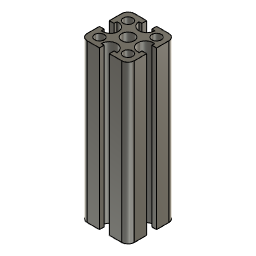
프로파일 2 v1 (Autodesk Fusion 360 design; units mm, degrees)
Autodesk Fusion 360 part; units mm, degrees
sketch "스케치1" plane through (0, 0, 0) normal (0, 0, 1) x (1, 0, 0)
  line L0 (-15, -11) -> (-15, -3.15)
  line L1 (-15, 3.15) -> (-15, 11)
  line L2 (15, 11) -> (15, 3.15)
  line L3 (15, -3.15) -> (15, -11)
  line L4 (-11, 15) -> (-3.15, 15)
  line L5 (3.15, 15) -> (11, 15)
  line L6 (11, -15) -> (3.15, -15)
  line L7 (-3.15, -15) -> (-11, -15)
  circle A0 centre (-9.075, 9.075) radius 3
  line L8 (-15.033, 3.15) -> (-12, 3.15)
  line L9 (-12, 9.075) -> (-12.075, 9.075)
  line L10 (-12, 4.9272) -> (-12, 3.15)
  circle A1 centre (0, 0) radius 4
  arc A2 (-15, 3.1902) -> (-15.033, 3.15) centre (-11.15, 0) ccw
  line L11 (-15.033, -3.15) -> (-12, -3.15)
  arc A3 (-15.033, -3.15) -> (-15, -3.1902) centre (-11.15, 0) ccw
  arc A4 (-12, -4.9272) -> (-12, 4.9272) centre (-11.15, 0) ccw
  line L12 (-5, 12) -> (-3.15, 12)
  arc A5 (-5, 12) -> (5, 12) centre (0, 12) ccw
  line L13 (-3.15, 15) -> (-3.15, 12)
  line L14 (3.15, 15) -> (3.15, 12)
  line L15 (3.15, 15) -> (3.15, 12)
  line L16 (12, 4.9272) -> (12, 3.15)
  arc A6 (12, 4.9272) -> (12, -4.9272) centre (11.15, 0) ccw
  line L17 (5, 12) -> (3.15, 12)
  line L18 (15, -11) -> (15, -3.15)
  arc A7 (15, -3.1902) -> (15.033, -3.15) centre (11.15, 0) ccw
  circle A8 centre (9.075, 9.075) radius 3
  line L19 (3.15, -15) -> (11, -15)
  arc A9 (15.033, 3.15) -> (15, 3.1902) centre (11.15, 0) ccw
  line L20 (15, 3.15) -> (15, 11)
  line L21 (-12, -3.15) -> (-12, -4.9272)
  line L22 (12, 3.15) -> (15, 3.15)
  line L23 (12, -3.15) -> (15, -3.15)
  line L24 (0, 0) -> (-20, 0)
  circle A10 centre (-9.075, -9.075) radius 3
  circle A11 centre (9.075, -9.075) radius 3
  line L25 (3.15, -15) -> (11, -15)
  line L26 (15, -11) -> (15, -3.15)
  line L27 (-15, -3.15) -> (-15, -11)
  line L28 (-15.033, -3.15) -> (-12, -3.15)
  arc A12 (5, -12) -> (-5, -12) centre (0, -12) ccw
  line L29 (15, -3.15) -> (15, -11)
  arc A13 (15, -3.1902) -> (15.033, -3.15) centre (11.15, 0) ccw
  arc A14 (-15.033, -3.15) -> (-15, -3.1902) centre (-11.15, 0) ccw
  line L30 (12, -4.9272) -> (12, -3.15)
  line L31 (12, -3.15) -> (15, -3.15)
  line L32 (-12, -4.9272) -> (-12, -3.15)
  line L33 (3.15, -15) -> (3.15, -12)
  line L34 (3.15, -15) -> (3.15, -12)
  line L35 (-5, -12) -> (-3.15, -12)
  line L36 (5, -12) -> (3.15, -12)
  line L37 (-3.15, -15) -> (-3.15, -12)
  line L38 (3.15, 12) -> (5, 12)
  line L39 (12, 4.9272) -> (12, 3.15)
  arc A15 (9.7416, 12) -> (12, 9.7416) centre (9.075, 9.075) ccw
  line L40 (-3.15, -12) -> (-3.15, -15)
  line L41 (3.15, -12) -> (3.15, -15)
  line L42 (3.15, -12) -> (3.15, -15)
  line L43 (3.15, -12) -> (5, -12)
  line L44 (3.15, -12) -> (5, -12)
  line L45 (12, -3.15) -> (12, -4.9272)
  line L46 (12, -4.9272) -> (12, -3.15)
  line L47 (12, -3.15) -> (12, -4.9272)
  arc A16 (6.075, -9.075) -> (8.4084, -6.15) centre (9.075, -9.075) ccw
  arc A17 (6.075, -9.075) -> (8.4084, -6.15) centre (9.075, -9.075) ccw
  arc A18 (6.075, -9.075) -> (8.4084, -6.15) centre (9.075, -9.075) ccw
  line L48 (-5, -12) -> (-3.15, -12)
  arc A19 (-8.4084, -6.15) -> (-12.075, -9.075) centre (-9.075, -9.075) ccw
  arc A20 (-11, 15) -> (-15, 11) centre (-11, 11) ccw
  arc A21 (15, 11) -> (11, 15) centre (11, 11) ccw
  arc A22 (11, -15) -> (15, -11) centre (11, -11) ccw
  arc A23 (-15, -11) -> (-11, -15) centre (-11, -11) ccw
  point P0 (15, -6.15)
  point P1 (15, -12)
  point P2 (12, 15)
  point P3 (9.075, -4.5491)
  point P4 (-9.075, -15)
  point P5 (0, -4)
  point P6 (-12, -15)
  point P7 (9.075, -15)
  point P8 (12, -15)
  dimension "d1" = 30
  dimension "d2" = 30
  dimension "d12" = 11.85
  dimension "d17" = 6
  dimension "d18" = 6
  dimension "d19" = 6
  dimension "d20" = 6
  dimension "d26" = 10
  dimension "d27" = 8
  dimension "d29" = 10
  dimension "d30" = 4
  constraint horizontal L4
  constraint vertical L2
  constraint horizontal L6
  constraint vertical L0
  constraint perpendicular L0 L8
  constraint perpendicular L0 L11
  constraint perpendicular L4 L14
  constraint coincident L7.start L6
  constraint coincident L3.start L2
  constraint coincident L1.start L8
  constraint collinear L0 L1
  constraint coincident L0.end L11
  constraint collinear L2 L3
  constraint collinear L4 L5
  constraint collinear L6 L7
  constraint coincident A0 L9.end
  constraint coincident L1 A2.start
  constraint coincident A1.centre L24.start
  constraint concentric A2 A3
  constraint coincident L0 A3.end
  constraint concentric A3 A4
  constraint horizontal L24
  constraint symmetric L2.end L24 L3.start
  constraint symmetric L1.start L24 L0.end
  constraint symmetric L4.end L24 L7.start
  constraint symmetric L5.start L24 L6.end
  constraint symmetric A0 L24 A10
  constraint symmetric L24 A15 A17
  constraint symmetric L8.end L24 L11.end
  constraint symmetric L12.end L24 L35.end
  constraint symmetric L14.end L24 L33.end
  constraint symmetric L10.start L24 A4.start
  constraint symmetric A2.start L24 A3.end
  constraint symmetric L8.start L24 L11.start
  constraint symmetric A2 L24 A14
  constraint symmetric L12.start L24 A12.end
  constraint symmetric A5 L24 A12
  constraint symmetric A5.end L24 A12.start
  constraint symmetric A9.end L24 A7.start
  constraint symmetric L16.start L24 A6.end
  constraint symmetric A9.start L24 A7.end
  constraint symmetric P2 L24 P8
  constraint symmetric L16.end L24 L23.start
  constraint symmetric A8 L24 A11
  constraint symmetric A9 L24 A13
  constraint tangent L4 A20
  constraint tangent L1 A20
  constraint tangent L20 A21
  constraint equal A20 A21
  constraint tangent L18 A22
  constraint tangent L6 A22
  constraint equal A20 A22
  constraint tangent L7 A23
  constraint tangent L0 A23
  constraint equal A20 A23
  measures "d1" distance of L0 L2
  measures "d2" distance of L4 L6
  measures "d12" distance of L4 L8
  measures "d17" diameter of A0
  measures "d18" diameter of A15
  measures "d19" diameter of A19
  measures "d20" diameter of A18
  measures "d26" diameter of A2
  measures "d27" diameter of A1
  measures "d29" diameter of A5
  measures "d30" radius of A20
extrude "돌출1" add sketch "스케치1" along normal blind 100 contours L0 L1 L2 L3 L4 L5 L6 L7 L8 L10 L11 A4 L12 A5 L13 L14 L15 L16 A6 L17 L18 L19 L20 L21 L22 L23 L25 L26 L27 L28 A12 L29 L30 L31 L32 L33 L34 L35 L36 L37 L38 L39 L40 L41 L42 L43 L44 L45 L46 L47 L48 A20 A21 A22 A23
